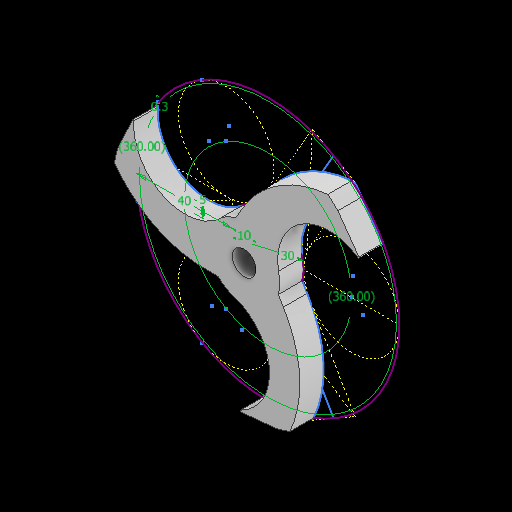
# Autodesk Inventor part: Combine mk2
Saved by Autodesk Inventor 2025 (Build 290162000, 162)
## iProperties
Created: 2024-09-10
Part Number: Combine mk2
Material: Generic
Document SubType Name: Modeling
Designer: Trevor
Density: 1 g/cm^3
Appearance: Default
Author: Trevor
Autodesk Inventor part; units mm, degrees
ref_plane "YZ Plane" through (0, 0, 0) normal (1, 0, 0) x (0, 1, 0)
ref_plane "XZ Plane" through (0, 0, 0) normal (0, 1, 0) x (-1, 0, 0)
ref_plane "XY Plane" through (0, 0, 0) normal (0, 0, 1) x (1, 0, 0)
sketch "Sketch1" plane through (0, 0, 0) normal (0, 0, 1) x (1, 0, 0)
  circle A0 centre (0, 0) radius 15
  circle A1 centre (0, 0) radius 55
  line L0 (15, 0) -> (55, 0) construction
  circle A2 centre (35, 0) radius 20 construction
  circle A3 centre (-17.5, 30.3109) radius 20 construction
  circle A4 centre (-17.5, -30.3109) radius 20 construction
  line L1 (0, 0) -> (-10.834, 10.3742)
  line L2 (0, 0) -> (27.5, -47.6314)
  line L3 (0, 0) -> (-55, 0) construction
  line L4 (0, 0) -> (27.5, 47.6314)
  line L5 (17.5, 30.3109) -> (27.5, 47.6314) construction
  line L6 (-1.4324, 18.1475) -> (18.5676, 52.7885) construction
  line L7 (18.5676, 52.7885) -> (36.4324, 42.4743) construction
  line L8 (36.4324, 42.4743) -> (16.4324, 7.8333) construction
  line L9 (16.4324, 7.8333) -> (-1.4324, 18.1475) construction
  line L10 (-1.4324, 18.1475) -> (36.4324, 42.4743) construction
  line L11 (18.5676, 52.7885) -> (16.4324, 7.8333) construction
  line L12 (-1.4891, -18.1802) -> (18.5109, -52.8212) construction
  line L13 (18.5109, -52.8212) -> (36.4891, -42.4416) construction
  line L14 (36.4891, -42.4416) -> (16.4891, -7.8006) construction
  line L15 (16.4891, -7.8006) -> (-1.4891, -18.1802) construction
  line L16 (-1.4891, -18.1802) -> (36.4891, -42.4416) construction
  line L17 (18.5109, -52.8212) -> (16.4891, -7.8006) construction
  line L18 (-55.0081, 10.3109) -> (-15, 10.3109) construction
  line L19 (-15, 10.3109) -> (-15, -10.3109) construction
  line L20 (-15, -10.3109) -> (-55.0081, -10.3109) construction
  line L21 (-55.0081, -10.3109) -> (-55.0081, 10.3109)
  line L22 (-55.0081, 10.3109) -> (-15, -10.3109) construction
  line L23 (-15, 10.3109) -> (-55.0081, -10.3109) construction
  line L24 (-39.1178, -2.5) -> (-30.8902, -2.5) construction
  line L25 (-30.8902, -2.5) -> (-30.8902, 2.5) construction
  line L26 (-30.8902, 2.5) -> (-39.1178, 2.5) construction
  line L27 (-39.1178, 2.5) -> (-39.1178, -2.5) construction
  line L28 (-39.1178, -2.5) -> (-30.8902, 2.5) construction
  line L29 (-30.8902, -2.5) -> (-39.1178, 2.5) construction
  line L30 (-55.0081, 10.3109) -> (-55.0081, -10.3109) construction
  line L31 (-55.0081, 10.3109) -> (-55.0081, -10.3109) construction
  circle A5 centre (0, 0) radius 5
  arc A6 (-54.3489, 9.3568) -> (-15, -10.3109) centre (-16.25, 36.3845) ccw
  arc A7 (-46.1231, 28.4056) -> (-10.834, 10.3742) centre (-24.6951, 26.7945) ccw
  line L32 (-15, -10.3109) -> (-10.8943, -10.3109)
  line L33 (-46.6952, 28.5525) -> (-54.5376, 11.3433)
  arc A8 (-46.1231, 28.4056) -> (-46.6952, 28.5525) centre (-46.4222, 28.4281) ccw
  arc A9 (-54.5376, 11.3433) -> (-54.3489, 9.3568) centre (-52.7176, 10.514) ccw
  arc A10 (17.4452, -52.9026) -> (19.0712, -51.7459) centre (17.2535, -50.9118) ccw
  line L34 (-1.3796, -54.7155) -> (17.4452, -52.9026)
  arc A11 (19.0712, -51.7459) -> (16.4295, -7.8349) centre (-23.3849, -32.2652) ccw
  arc A12 (-1.5384, -54.1465) -> (-3.5673, -14.5696) centre (-10.8572, -34.7838) ccw
  circle A13 centre (0, 0) radius 15
  line L35 (16.4295, -7.8349) -> (14.3766, -4.2793)
  arc A14 (-1.5384, -54.1465) -> (-1.3796, -54.7155) centre (-1.4083, -54.4169) ccw
  arc A15 (37.0924, 41.5593) -> (35.2776, 42.3891) centre (35.4642, 40.3978) ccw
  line L36 (48.0748, 26.163) -> (37.0924, 41.5593)
  arc A16 (35.2776, 42.3891) -> (-1.4295, 18.1458) centre (39.6349, -4.1193) ccw
  arc A17 (47.6615, 25.741) -> (14.4013, 4.1954) centre (35.5523, 7.9893) ccw
  circle A18 centre (0, 0) radius 15
  line L37 (-1.4295, 18.1458) -> (-3.4823, 14.5902)
  arc A19 (47.6615, 25.741) -> (48.0748, 26.163) centre (47.8305, 25.9888) ccw
  point P0 (-27.5, 47.6314)
  point P1 (-27.5, -47.6314)
  point P2 (17.5, -30.3109)
  point P3 (-35.004, 0)
  point P4 (-45.8939, 30.3109)
  point P5 (-7.5, 12.9904)
  point P6 (-7.5, -12.9904)
  point P7 (-52.9855, 14.7493)
  point P8 (-54.2274, 9.1864)
  point P9 (-3.5673, -14.5696)
  point P10 (13.7195, -53.2614)
  point P11 (19.1581, -51.5555)
  point P12 (14.4013, 4.1954)
  point P13 (39.266, 38.5121)
  point P14 (35.0693, 42.3691)
  dimension "d0" = 30
  dimension "d1" = 40
  dimension "d4" = 360
  dimension "d6" = 5
  dimension "d11" = 10
  dimension "d14" = 0.3
  dimension "d22" = 360
  constraints: 76 end point, 40 point on circle, 17 centre point, 9 midpoint, 9 parallel, 6 point on line, 4 perpendicular, 4 tangent, 3 coincident, 3 horizontal, 1 horizontal alignment, 80 other
  measures "d0" diameter of A0
  measures "d1" radial gap between concentric circles of A0 A1
  measures "d6" distance of L25.end L24.end
  measures "d11" radial gap between concentric circles of A0 A5
  measures "d14" radius of A8
extrude "Extrusion1" add sketch "Sketch1" along normal blind 10 contours A0 L2 A5 L4 | A0 L4 A16 A1 L36 A19 A17 | L35 A11 L2 A0 | L4 A5 L1 A0 | A0 L37 A16 L4 | L2 A11 A1 L34 A14 A12 A0 | A0 L1 A5 L2 | A0 L32 A6 A1 L33 A8 A7
body "Solid1"
